hotend_holder_induction_probe_12 (Autodesk Fusion 360 design; units mm, degrees)
Autodesk Fusion 360 part; units mm, degrees
sketch "Sketch1" plane through (0, 0, 0) normal (0, 1, 0) x (1, 0, 0)
  line L0 (-27, 25) -> (-27, 20)
  line L1 (-27, 20) -> (-15, 20)
  line L2 (-15, 20) -> (-15, 0)
  line L3 (-15, 0) -> (15, 0)
  line L4 (15, 0) -> (15, 20)
  line L5 (15, 20) -> (27, 20)
  line L6 (27, 20) -> (27, 25)
  line L7 (27, 25) -> (-27, 25)
  dimension "d1" = 54
  dimension "d2" = 12
  dimension "d3" = 30
  dimension "d4" = 5
  dimension "d5" = 20
  constraint vertical L0
  constraint perpendicular L0 L1
  constraint perpendicular L1 L2
  constraint perpendicular L2 L3
  constraint perpendicular L1 L4
  constraint perpendicular L2 L5
  constraint perpendicular L5 L6
  constraint horizontal L7
  constraint midpoint origin L3
  constraint collinear L1 L5
  measures "d1" distance of L0.start L6.end
  measures "d2" distance of L0.end L1.end
  measures "d3" distance of L2.end L3.end
  measures "d4" distance of L0.start L0.end
  measures "d5" distance of L1.end L2.end
extrude "Extrude1" add sketch "Sketch1" along normal blind 69 makes body 1
sketch "Sketch2" plane through (0, 0, 0) normal (0, 0, 1) x (1, 0, 0)
  line L0 (-15, 0) -> (15, 0)
  line L1 (15, 0) -> (15, 69)
  line L2 (15, 69) -> (-15, 69)
  line L3 (-15, 69) -> (-15, 0)
  line L4 (-15, 69) -> (15, 69)
  line L5 (15, 69) -> (15, 42)
  line L6 (15, 42) -> (-15, 42)
  line L7 (-15, 42) -> (-15, 69)
  dimension "d8" = 42
  constraint horizontal L4
  constraint vertical L5
  constraint horizontal L6
  constraint vertical L7
  constraint coincident L1 L5.end
  constraint coincident L2.end L3.start
  measures "d8" distance of L0 L6
extrude "Extrude2" cut sketch "Sketch2" against normal blind 12 contours L1 L2 L3 L4 L5 L6 L7 bodies 1
sketch "Sketch3" plane through (0, 0, 0) normal (1, 0, 0) x (0, 0, -1)
  line L0 (0, 0) -> (0, 42)
  line L1 (20, 0) -> (0, 0)
  line L2 (11.25, 0) -> (11.25, 30)
  line L3 (11.25, 30) -> (8.1, 30)
  line L4 (8.1, 30) -> (8.1, 33.1)
  line L5 (8.1, 33.1) -> (6.1, 33.1)
  line L6 (6.1, 33.1) -> (6.1, 38.9)
  line L7 (6.1, 38.9) -> (8.1, 38.9)
  line L8 (8.1, 38.9) -> (8.1, 42)
  line L9 (0, 42) -> (12, 42)
  dimension "d11" = 11.25
  dimension "d12" = 8.1
  dimension "d13" = 6.1
  dimension "d14" = 30
  dimension "d15" = 3.1
  dimension "d16" = 5.8
  constraint coincident L1 L2.start
  constraint perpendicular L1 L2
  constraint perpendicular L0 L3
  constraint perpendicular L3 L4
  constraint perpendicular L4 L5
  constraint perpendicular L3 L6
  constraint perpendicular L6 L7
  constraint perpendicular L7 L8
  constraint coincident L8.end L9
  constraint collinear L4 L8
  measures "d11" distance of L0 L2
  measures "d12" distance of L0 L8
  measures "d13" distance of L0 L6
  measures "d14" distance of L2.start L2.end
  measures "d15" distance of L3.end L4.end
  measures "d16" distance of L5.end L6.end
sketch "Sketch4" plane through (-15, 0, 0) normal (-1, 0, 0) x (0, 0, 1)
  line L0 (-12, 42) -> (-12, 69)
  line L1 (-12, 69) -> (-20, 69)
  line L2 (-20, 69) -> (-20, 0)
  line L3 (-20, 0) -> (0, 0)
  line L4 (0, 0) -> (0, 42)
  line L5 (0, 42) -> (-12, 42)
  circle A0 centre (0, 17) radius 14
  dimension "d18" = 28
  dimension "d19" = 17
  constraint coincident L4 A0.centre
  measures "d18" diameter of A0
  measures "d19" distance of L3.end A0.centre
sketch "Sketch6" plane through (0, 0, -20) normal (0, 0, 1) x (1, 0, 0)
  line L0 (15, 0) -> (27, 0)
  line L1 (27, 0) -> (27, 69)
  line L2 (27, 69) -> (15, 69)
  line L3 (15, 69) -> (15, 0)
  circle A0 centre (27, 23) radius 5
  dimension "d25" = 10
  dimension "d26" = 23
  constraint coincident L1 A0.centre
  measures "d25" diameter of A0
  measures "d26" distance of L0.end A0.centre
extrude "Extrude5" cut sketch "Sketch6" against normal through all contours L1 A0 picked at (25.338, 23.1246) bodies 1
sketch "Sketch7" plane through (0, 0, 0) normal (0, 0, 1) x (1, 0, 0)
  line L0 (15, 42) -> (-15, 42)
  line L1 (-15, 42) -> (-15, 0)
  line L2 (-15, 42) -> (15, 42)
  line L3 (15, 42) -> (15, 0)
  line L4 (15, 0) -> (-15, 0)
  line L5 (-15, 0) -> (-15, 42)
  line L6 (15, 0) -> (15, 42)
  line L7 (-15, 0) -> (15, 0)
  point P0 (15, 0)
  constraint horizontal L2
  constraint vertical L3
  constraint horizontal L4
  constraint vertical L5
  constraint coincident L0.end L1.start
  constraint coincident P0 L3.end
extrude "Extrude1'" add sketch "Sketch7" along normal blind 20 separate body makes body 2 in component "Component"
revolve "Revolve1" cut sketch "Sketch3" angle 360 about axis through (0, 0, 0) along (0, 1, 0) bodies 1
revolve "Revolve1'" cut sketch "Sketch3" angle 360 about axis through (0, 0, 0) along (0, 1, 0) bodies 2 in component "Component"
extrude "Extrude3" cut sketch "Sketch4" against normal through all contours L4 A0 | L4 A0 bodies 1
extrude "Extrude2'" cut sketch "Sketch4" against normal through all contours L4 A0 | L4 A0 bodies 2 in component "Component"
sketch "Sketch8" plane through (0, 0, 20) normal (0, 0, 1) x (1, 0, 0)
  line L0 (-15, 42) -> (-15, 0)
  line L1 (-15, 0) -> (15, 0)
  line L2 (15, 0) -> (15, 42)
  line L3 (15, 42) -> (-15, 42)
  line L4 (15, 10.1036) -> (32.5, 0)
  line L5 (15, 15.8771) -> (35, 4.3301)
  line L6 (35.8546, 2.85) -> (34.2091, 0)
  line L7 (34.2091, 0) -> (35.8546, -2.85)
  line L8 (35.8546, -2.85) -> (39.1454, -2.85)
  line L9 (39.1454, -2.85) -> (40.7909, 0)
  line L10 (40.7909, 0) -> (39.1454, 2.85)
  line L11 (39.1454, 2.85) -> (35.8546, 2.85)
  line L12 (42.5, 0) -> (40, 4.3301)
  line L13 (40, 4.3301) -> (35, 4.3301)
  line L14 (35, 4.3301) -> (32.5, 0)
  line L15 (32.5, 0) -> (35, -4.3301)
  line L16 (35, -4.3301) -> (40, -4.3301)
  line L17 (40, -4.3301) -> (42.5, 0)
  circle A0 centre (-5.5, 38) radius 2
  circle A1 centre (37.5, 0) radius 1.6
  point P0 (37.5, 0)
  point P1 (37.5, 0)
  dimension "d32" = 5.7
  dimension "d34" = 60
  dimension "d35" = 5
  dimension "d36" = 3.2
  dimension "d37" = 4
  dimension "d38" = 43
  dimension "d39" = 38
  dimension "d40" = 4
  dimension "d41" = 9.5
  constraint coincident L2 L4.start
  constraint coincident L2 L5.start
  constraint coincident P1 P0
  constraint parallel L4 L5
  constraint perpendicular L4 L14
  constraint parallel L7 L15
  measures "d32" distance of L7 L10
  measures "d34" angle of L2 L4
  measures "d35" distance of L4 L5
  measures "d36" diameter of A1
  measures "d37" diameter of A0
  measures "d38" horizontal distance of A0.centre P1
  measures "d39" vertical distance of A0.centre P1
  measures "d40" distance of L3 A0.centre
  measures "d41" distance of L0 A0.centre
extrude "Extrude3'" add sketch "Sketch8" against normal blind 3 contours L2 L4 L5 L14 | L12 L13 L14 L15 L16 L17 | L6 L7 L8 L9 L10 L11 bodies 2 in component "Component"
extrude "Extrude4" add sketch "Sketch8" against normal blind 1 from surface at -3 contours L12 L13 L14 L15 L16 L17 bodies 2 in component "Component"
extrude "Extrude5'" cut 1 faces at (39.5861, -1.2504, 17) along direction (0, 0, 1) blind 1 on bodies 2 bodies 2 in component "Component"
extrude "Extrude6" cut sketch "Sketch8" against normal blind 10 contours A0 bodies 2 in component "Component"
sketch "Sketch9" plane through (0, 0, 20) normal (0, 0, 1) x (1, 0, 0)
  circle A0 centre (-5.5, 38) radius 2
  circle A1 centre (37.5, 0) radius 1.6
  line L0 (-15, 42) -> (-15, 0)
  line L1 (-15, 0) -> (15, 0)
  line L2 (15, 0) -> (15, 10.1036)
  line L3 (15, 10.1036) -> (32.5, 0)
  line L4 (32.5, 0) -> (35, -4.3301)
  line L5 (35, -4.3301) -> (40, -4.3301)
  line L6 (40, -4.3301) -> (42.5, 0)
  line L7 (42.5, 0) -> (40, 4.3301)
  line L8 (40, 4.3301) -> (35, 4.3301)
  line L9 (35, 4.3301) -> (15, 15.8771)
  line L10 (15, 15.8771) -> (15, 42)
  line L11 (15, 42) -> (-15, 42)
  line L12 (-15, 0) -> (15, 0)
  line L13 (15, 0) -> (15, -6.5)
  line L14 (15, -6.5) -> (-19.1, -6.5)
  line L15 (-19.1, -6.5) -> (-19.1, 0)
  circle A2 centre (-14.5, -3) radius 2
  line L16 (-19.1, 0) -> (-15, 0)
  dimension "d52" = 4
  dimension "d53" = 4.6
  dimension "d62" = 14.5
  dimension "d63" = 6.5
  dimension "d64" = 3
  constraint horizontal L12
  constraint vertical L13
  constraint horizontal L14
  constraint vertical L15
  constraint coincident L1.end L2.start
  constraint coincident L0.end L1.start
  constraint perpendicular L0 L16
  measures "d52" diameter of A2
  measures "d53" distance of L15 A2.centre
  measures "d62" horizontal distance of origin A2.centre
  measures "d63" distance of L1.end L13.end
  measures "d64" distance of L12 A2.centre
extrude "Extrude7" add sketch "Sketch9" against normal blind 7 contours L1 L12 L13 L14 L15 L16 bodies 2 in component "Component"
sketch "Sketch10" plane through (-15, 0, 0) normal (-1, 0, 0) x (0, 0, 1)
  arc A0 (0, 31) -> (0, 3) centre (0, 17) ccw
  line L0 (0, 31) -> (0, 42)
  line L1 (0, 42) -> (-12, 42)
  line L2 (-12, 42) -> (-12, 69)
  line L3 (-12, 69) -> (-20, 69)
  line L4 (-20, 69) -> (-20, 0)
  line L5 (-20, 0) -> (0, 0)
  line L6 (0, 0) -> (0, 3)
  circle A1 centre (-15.8, 36.2) radius 2
  circle A2 centre (-15.8, 4.2) radius 2
  circle A3 centre (16.2, 4.2) radius 2
  dimension "d66" = 4
  dimension "d67" = 32
  dimension "d68" = 32
  dimension "d70" = 15.8
  dimension "d71" = 4.2
  constraint equal A2 A3
  constraint horizontal A2.centre A3.centre
  constraint vertical A1.centre A2.centre
  measures "d66" diameter of A2
  measures "d67" distance of A1.centre A2.centre
  measures "d68" horizontal distance of A2.centre A3.centre
  measures "d70" horizontal distance of L5.end A2.centre
  measures "d71" distance of L5 A2.centre
extrude "Extrude6'" cut sketch "Sketch10" against normal blind 10 contours A1 | A2 | A3 bodies 1
extrude "Extrude8" cut sketch "Sketch10" against normal blind 10 contours A1 | A2 | A3 bodies 2 in component "Component"
sketch "Sketch11" plane through (0, 0, 13) normal (0, 0, -1) x (-1, 0, 0)
  circle A0 centre (14.5, -3) radius 2
  line L0 (19.1, 0) -> (15, 0)
  line L1 (15, 0) -> (-15, 0)
  line L2 (-15, 0) -> (-15, -6.5)
  line L3 (-15, -6.5) -> (19.1, -6.5)
  line L4 (19.1, -6.5) -> (19.1, 0)
  line L5 (9.5, -6.5) -> (9.5, 0)
  dimension "d76" = 5
  constraint coincident L3 L5.start
  constraint coincident L1 L5.end
  constraint perpendicular L1 L5
  measures "d76" distance of A0.centre L5
extrude "Extrude9" cut sketch "Sketch11" against normal blind 4 contours L1 L2 L3 L5 bodies 2 in component "Component"
sketch "Sketch12" plane through (0, 0, 20) normal (0, 0, 1) x (1, 0, 0)
  circle A0 centre (-14.5, -3) radius 2
  circle A1 centre (-5.5, 38) radius 2
  circle A2 centre (37.5, 0) radius 1.6
  line L0 (-15, 42) -> (-15, 0)
  line L1 (-15, 0) -> (-19.1, 0)
  line L2 (-19.1, 0) -> (-19.1, -6.5)
  line L3 (-19.1, -6.5) -> (15, -6.5)
  line L4 (15, -6.5) -> (15, 10.1036)
  line L5 (15, 10.1036) -> (32.5, 0)
  line L6 (32.5, 0) -> (35, -4.3301)
  line L7 (35, -4.3301) -> (40, -4.3301)
  line L8 (40, -4.3301) -> (42.5, 0)
  line L9 (42.5, 0) -> (40, 4.3301)
  line L10 (40, 4.3301) -> (35, 4.3301)
  line L11 (35, 4.3301) -> (15, 15.8771)
  line L12 (15, 15.8771) -> (15, 42)
  line L13 (15, 42) -> (-15, 42)
  circle A3 centre (-11, 36.5) radius 1.6
  circle A4 centre (11, 36.5) radius 2
  circle A5 centre (11, 36.5) radius 1.6
  circle A6 centre (-11, 36.5) radius 2
  line L14 (-15, 31) -> (-8.1, 31)
  line L15 (-8.1, 31) -> (-8.1, 33.1)
  line L16 (-8.1, 33.1) -> (-6.1, 33.1)
  line L17 (-6.1, 33.1) -> (-6.1, 38.9)
  line L18 (-6.1, 38.9) -> (-8.1, 38.9)
  line L19 (-8.1, 38.9) -> (-8.1, 42)
  line L20 (-8.1, 42) -> (-15, 42)
  line L21 (-15, 42) -> (-15, 31)
  circle A7 centre (-11, 36.5) radius 3.1
  circle A8 centre (11, 36.5) radius 3.1
  point P0 (-15, 36.5)
  dimension "d79" = 3.2
  dimension "d80" = 4
  dimension "d81" = 4
  dimension "d82" = 4
  dimension "d87" = 6.2
  constraint concentric A4 A5
  constraint concentric A3 A6
  constraint equal A4 A6
  constraint equal A3 A5
  constraint midpoint L21 P0
  constraint horizontal A3.centre P0
  constraint horizontal A3.centre A4.centre
  constraint concentric A3 A7
  constraint concentric A5 A8
  constraint equal A7 A8
  measures "d79" diameter of A3
  measures "d80" diameter of A6
  measures "d81" distance of A3.centre L21
  measures "d82" distance of L12 A4.centre
  measures "d87" diameter of A7
extrude "Extrude10" cut sketch "Sketch12" against normal through all contours A3 | A5 bodies 2 in component "Component"
extrude "Extrude7'" cut sketch "Sketch12" against normal blind 10 from surface at -20 contours A3 | A4 | A5 | A6 bodies 1
extrude "Extrude11" cut sketch "Sketch12" against normal blind 3.5 contours A4 | A6 | A7 | A8 bodies 2 in component "Component"
sketch "Sketch13" plane through (0, 0, 0) normal (0, -1, 0) x (1, 0, 0)
  arc A0 (-11.25, 0) -> (11.25, 0) centre (0, 0) ccw
  line L0 (-11.25, 0) -> (-15, 0)
  line L1 (-15, 0) -> (-15, -20)
  line L2 (-15, -20) -> (-27, -20)
  line L3 (-27, -20) -> (-27, -25)
  line L4 (-27, -25) -> (27, -25)
  line L5 (27, -25) -> (27, -20)
  line L6 (27, -20) -> (15, -20)
  line L7 (15, -20) -> (15, 0)
  line L8 (15, 0) -> (11.25, 0)
  circle A1 centre (30, -10) radius 6.1
  line L9 (27, -20) -> (27, -19.5394)
  circle A2 centre (30, -10) radius 10
  circle A3 centre (32.5, -17.0711) radius 17.5
  line L10 (27, -20) -> (30, -20)
  dimension "d90" = 12.2
  dimension "d91" = 20
  dimension "d92" = 10
  dimension "d93" = 15
  dimension "d121" = 35
  constraint concentric A1 A2
  constraint coincident L5.end L6.start
  constraint perpendicular L6 L9
  constraint coincident L9.end A2
  constraint tangent A2 A3
  constraint tangent L7 A3
  constraint coincident A2 L10.end
  constraint tangent A2 L10
  measures "d90" diameter of A1
  measures "d91" diameter of A2
  measures "d92" distance of L6 A1.centre
  measures "d93" distance of L7 A1.centre
  measures "d121" diameter of A3
extrude "Extrude8'" add sketch "Sketch13" against normal blind 8 from surface at -8 contours L6 L7 A3 | L6 L9 A2 A3 | A2 | L9 A2 L10 bodies 1
sketch "Sketch14" plane through (0, 0, -25) normal (0, 0, -1) x (-1, 0, 0)
  arc A0 (-27, 18) -> (-27, 28) centre (-27, 23) ccw
  line L0 (-27, 18) -> (-27, 0)
  line L1 (-27, 0) -> (27, 0)
  line L2 (27, 0) -> (27, 69)
  line L3 (27, 69) -> (-27, 69)
  line L4 (-27, 69) -> (-27, 28)
  circle A1 centre (-23, 48) radius 1.6
  circle A2 centre (23, 48) radius 1.6
  circle A3 centre (0, 26) radius 1.6
  line L5 (-23, 48) -> (23, 48) construction
  circle A4 centre (-23, 48) radius 3.1
  circle A5 centre (0, 26) radius 3.1
  circle A6 centre (23, 48) radius 3.1
  point P0 (0, 48)
  dimension "d97" = 46
  dimension "d98" = 48
  dimension "d99" = 26
  dimension "d100" = 3.2
  dimension "d101" = 6.2
  constraint vertical origin A3.centre
  constraint coincident A1.centre L5.start
  constraint coincident A2.centre L5.end
  constraint perpendicular L2 L5
  constraint midpoint L5 P0
  constraint vertical origin P0
  constraint equal A1 A2
  constraint equal A2 A3
  constraint concentric A3 A5
  constraint concentric A2 A6
  constraint equal A4 A6
  constraint equal A5 A6
  measures "d97" distance of A1.centre A2.centre
  measures "d98" distance of L1 A1.centre
  measures "d99" vertical distance of origin A3.centre
  measures "d100" diameter of A1
  measures "d101" diameter of A4
extrude "Extrude9'" cut sketch "Sketch14" against normal through all contours A1 | A2 | A3 bodies 1
extrude "Extrude10'" cut sketch "Sketch14" against normal through all from surface at -2 contours A4 | A5 | A6 bodies 1
sketch "Sketch15" plane through (0, 0, -20) normal (0, 0, 1) x (1, 0, 0)
  line L0 (15, 8) -> (15, 0)
  line L1 (15, 0) -> (27, 0)
  line L2 (27, 0) -> (27, 8)
  circle A0 centre (15, 8) radius 5
  circle A1 centre (15, 16) radius 5
  line L3 (10, 16) -> (10, 8)
  line L4 (40, 16) -> (26.6667, 16)
  line L5 (27, 8) -> (15, 8)
  line L6 (15, 8) -> (15, 16)
  line L7 (15, 16) -> (26.6667, 16)
  dimension "d105" = 10
  constraint coincident L0.start A0.centre
  constraint equal A0 A1
  constraint coincident A1 L3.start
  constraint coincident A0 L3.end
  constraint tangent A0 L3
  constraint tangent A1 L3
  constraint coincident A1.centre L6.end
  constraint perpendicular L5 L6
  constraint coincident L4.end L7.end
  constraint perpendicular L6 L7
  measures "d105" diameter of A1
extrude "Extrude11'" cut sketch "Sketch15" along normal blind 28 from surface at 5 contours L0 A0 L5 | L0 A0 A1 L6 | A0 A1 L6 | A0 A1 L3 | A0 A1 L6 L7 picked at (14.7861, 11.6805) picked at (13.0389, 14.3) bodies 1
sketch "Sketch16" plane through (0, 0, 0) normal (0, -1, 0) x (1, 0, 0)
  arc A0 (-11.25, 0) -> (11.25, 0) centre (0, 0) ccw
  line L0 (-11.25, 0) -> (-15, 0)
  line L1 (-15, 0) -> (-15, -20)
  line L2 (-15, -20) -> (-27, -20)
  line L3 (-27, -20) -> (-27, -25)
  line L4 (-27, -25) -> (27, -25)
  line L5 (27, -25) -> (27, -20)
  line L6 (27, -20) -> (15, -20)
  line L7 (15, -20) -> (15, 0)
  line L8 (15, 0) -> (11.25, 0)
  line L9 (-19, -20) -> (-19, -22)
  line L10 (-19, -22) -> (18, -22)
  line L11 (18, -22) -> (18, -20)
  line L12 (15, -18) -> (-15, -18)
  dimension "d109" = 4
  dimension "d110" = 2
  dimension "d111" = 4
  dimension "d112" = 3
  constraint coincident L2 L9.start
  constraint perpendicular L2 L9
  constraint perpendicular L9 L10
  constraint coincident L6 L11.end
  constraint perpendicular L6 L11
  constraint coincident L7 L12.start
  constraint coincident L1 L12.end
  constraint perpendicular L1 L12
  measures "d109" distance of L10 L12
  measures "d110" distance of L2 L10
  measures "d111" distance of L1 L9
  measures "d112" distance of L7 L11
fillet "Fillet3" radius 2.5 18 edges at (15, 42, -6) (-15, 55.5, -12) (15, 55.5, -12) (0, 69, -12) (-15, 42, -6) (-15, 69, -16) (15, 69, -16) (21, 69, -20) (27, 48.5, -20) (27, 69, -22.5) (27, 4, -20) (27, 0, -22.5) (21, 0, -20) (-27, 34.5, -20) (-27, 0, -22.5) (-27, 69, -22.5) (-21, 69, -20) (-21, 0, -20) on bodies 1
fillet "Fillet1" radius 2.5 4 edges at (15, 15.8771, 18.5) (15, 10.1036, 18.5) (15, 42, 10) (-15, 42, 10) on bodies 2 in component "Component"
fillet "Fillet2" radius 2 7 edges at (35, 4.3301, 18.5) (40, 4.3301, 18) (40, -4.3301, 18) (42.5, 0, 18) (35, -4.3301, 18) (32.5, 0, 18.5) (33.75, 2.1651, 17) on bodies 2 in component "Component"
extrude "Extrude14" add 1 faces at (28, 10.6667, -20) along direction (0, 0, -1) up to surface (5 mm away) on bodies 1 bodies 1
fillet "Fillet4" radius 3 1 edges at (30, 12, -20) on bodies 1
chamfer "Chamfer1" distance 4 angle 45 1 edges at (-15, 17, -14) on bodies 1
chamfer "Chamfer1'" distance 4 angle 45 1 edges at (-15, 17, 14) on bodies 2 in component "Component"
component "Component" placed x (1, 0, 0) y (0, 1, 0) z (0, 0, 1) at (0, 0, 0)
equation "d11 = ( 22.5 / 2 ) * 1 mm"
equation "d68 = d67"
equation "d70 = d68 / 2 - 0.2 mm"
equation "d82 = d81"
equation "d110 = d109 / 2"
